Autodesk Fusion 360 part; units mm, degrees
(part 4 of 4)
sketch "wood table" plane through (0, 0, -15.7932) normal (0, 0, -1) x (1, 0, 0)
  ellipse E0 centre (209.6118, -1.3037) end of major axis (209.6118, -4.1144) minor radius 2.8
  ellipse E1 centre (85.8572, -1.3037) end of major axis (85.8572, -4.1144) minor radius 2.8
  ellipse E2 centre (360.0651, -4.2438) end of major axis (360.0651, -7.0545) minor radius 2.8
  ellipse E3 centre (-5.0702, -4.2438) end of major axis (-5.0702, -7.0545) minor radius 2.8
  ellipse E4 centre (85.8572, -121.7862) end of major axis (85.8572, -124.5969) minor radius 2.8
  ellipse E5 centre (209.6118, -121.7862) end of major axis (209.6118, -124.5969) minor radius 2.8
  ellipse E6 centre (-5.0702, -118.846) end of major axis (-5.0702, -121.6567) minor radius 2.8
  ellipse E7 centre (360.0651, -118.846) end of major axis (360.0651, -121.6567) minor radius 2.8
  ellipse E8 centre (147.7321, -2.5781) end of major axis (147.7321, 13.483) minor radius 16 (150.5116, 13.2388) -> (144.9524, 13.2388) ccw
  line L0 (144.9524, 13.2388) -> (109.481, 6.9571)
  line L1 (109.481, 6.9571) -> (85.5071, 2.7116)
  line L2 (85.5071, 2.7116) -> (2.0009, 2.7116)
  ellipse E9 centre (2.0009, -11.3419) end of major axis (2.0009, 2.7116) minor radius 14 (2.0009, 2.7116) -> (-11.9991, -11.3419) ccw
  line L3 (-11.9991, -11.3419) -> (-11.9991, -111.748)
  ellipse E10 centre (2.0009, -111.748) end of major axis (2.0009, -125.8014) minor radius 14 (-11.9991, -111.748) -> (2.0009, -125.8014) ccw
  line L4 (2.0009, -125.8014) -> (352.994, -125.8014)
  ellipse E11 centre (352.994, -111.748) end of major axis (352.994, -125.8014) minor radius 14 (352.994, -125.8014) -> (366.994, -111.748) ccw
  line L5 (366.994, -111.748) -> (366.994, -11.3419)
  ellipse E12 centre (352.994, -11.3419) end of major axis (352.994, 2.7116) minor radius 14 (366.994, -11.3419) -> (352.994, 2.7116) ccw
  line L6 (352.994, 2.7116) -> (209.9619, 2.7116)
  line L7 (209.9619, 2.7116) -> (150.5116, 13.2388)
  line L8 (-11.9991, -61.5449) -> (366.994, -61.5449) construction
  line L9 (787.0975, -290.1449) -> (-432.1025, -290.1449)
  line L10 (-432.1025, -290.1449) -> (-432.1025, 167.0551)
  line L11 (-432.1025, 167.0551) -> (787.0975, 167.0551)
  line L12 (787.0975, 167.0551) -> (787.0975, -290.1449)
  line L13 (787.0975, -290.1449) -> (-432.1025, 167.0551) construction
  line L14 (-432.1025, -290.1449) -> (787.0975, 167.0551) construction
  point P0 (177.4975, -61.5449)
  dimension "d176" = 1219.2
  dimension "d177" = 457.2
  constraint midpoint L3 L8.start
  constraint midpoint L5 L8.end
  constraint horizontal L9
  constraint perpendicular L9 L10
  constraint parallel L9 L11
  constraint parallel L10 L12
  constraint coincident L13 P0
  constraint coincident L14 P0
  constraint midpoint L8 P0
  measures "d176" distance of L10.end L11.end
  measures "d177" distance of L9.end L10.end
extrude "Extrude21" add sketch "wood table" along normal blind 31.75 separate body contours E0 | E1 | E2 | E3 | E4 | E5 | E6 | E7 | E8 L0 L1 L2 E9 L3 E10 L4 E11 L5 E12 L6 L7 | L9 L10 L11 L12 makes body 4
hidden bodies 4
equation "d97 = ( 3.25 / 2 ) * 1 mm"
equation "d129 = ( 5 / 3 ) * 1 mm"
equation "d130 = ( 5 / 3 ) * 1 mm"
named bodies: "plate", "top", "bottom", "table"
